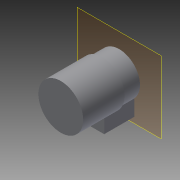
# Autodesk Inventor part: dragonFlyLens
Saved by Autodesk Inventor 2013 (Build 170138000, 138)
## iProperties
Created: 2014-07-04
Part Number: dragonFlyLens
Material: Generic
Document SubType Name: Modeling
Designer: Nano
Density: 1 g/cm^3
Author: Nano
Autodesk Inventor part; units mm, degrees
ref_plane "YZ Plane" through (0, 0, 0) normal (1, 0, 0) x (0, 1, 0)
ref_plane "XZ Plane" through (0, 0, 0) normal (0, 1, 0) x (-1, 0, 0)
ref_plane "XY Plane" through (0, 0, 0) normal (0, 0, 1) x (1, 0, 0)
ref_plane "Work Plane1" through (0, 0, 0) normal (0, 0, 1) x (1, 0, 0)
sketch "Sketch1" plane through (0, 0, 0) normal (0, 0, 1) x (1, 0, 0)
  circle A0 centre (0, 0) radius 18.669
  line L0 (13.462, -27.1587) -> (-13.462, -27.1587)
  line L1 (-13.462, -27.1587) -> (-13.462, -12.9347)
  line L2 (-13.462, -12.9347) -> (13.462, -12.9347)
  line L3 (13.462, -12.9347) -> (13.462, -27.1587)
  dimension "d0" = 37.338
  dimension "d1" = 26.924
  dimension "d2" = 14.224
  constraints: 8 end point, 2 parallel, 2 point on circle, 1 centre point, 1 horizontal, 1 perpendicular, 1 other
  measures "d0" diameter of A0
  measures "d1" distance of L1.end L2.end
  measures "d2" distance of L0.end L1.end
extrude "Extrusion1" add sketch "Sketch1" along normal blind 15.24
sketch "Sketch2" plane through (0, 0, 15.24) normal (0, 0, 1) x (1, 0, 0)
  line L0 (-13.462, -12.9347) -> (-13.462, -27.1587) projected
  line L1 (-13.462, -27.1587) -> (13.462, -27.1587) projected
  line L2 (13.462, -27.1587) -> (13.462, -12.9347) projected
  arc A0 (13.462, -12.9347) -> (-13.462, -12.9347) centre (0, 0) ccw projected
  circle A1 centre (0, 0) radius 20.066
  dimension "d5" = 40.132
  constraints: 1 centre point
  measures "d5" diameter of A1
extrude "Extrusion2" add sketch "Sketch2" along normal blind 11.684
sketch "Sketch3" plane through (0, 0, 26.924) normal (0, 0, 1) x (1, 0, 0)
  circle A0 centre (0, 0) radius 20.066
  constraints: 1 centre point
extrude "Extrusion3" add sketch "Sketch3" along normal blind 25.4
body "Solid1"
